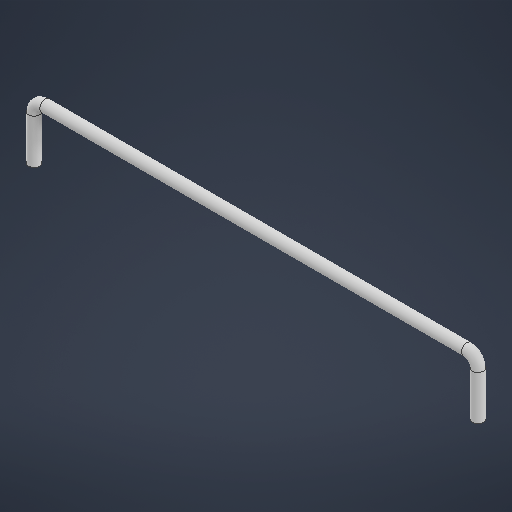
# Autodesk Inventor part: drut
Saved by Autodesk Inventor 2026.2 (Build 302298000, 298)
## iProperties
Created: 2025-12-09
Part Number: drut
Material: Generic
Document SubType Name: Modeling
Designer: janek
Density: 1 g/cm^3
Appearance: Default
Author: janek
Autodesk Inventor part; units mm, degrees
ref_plane "YZ Plane" through (0, 0, 0) normal (1, 0, 0) x (0, 1, 0)
ref_plane "XZ Plane" through (0, 0, 0) normal (0, 1, 0) x (-1, 0, 0)
ref_plane "XY Plane" through (0, 0, 0) normal (0, 0, 1) x (1, 0, 0)
sketch "Sketch1" plane through (0, 0, 0) normal (0, 0, 1) x (1, 0, 0)
  line L0 (0, 0) -> (0, 8)
  line L1 (2, 10) -> (78, 10)
  line L2 (80, 8) -> (80, 0)
  arc A0 (2, 10) -> (0, 8) centre (2, 8) ccw
  arc A1 (80, 8) -> (78, 10) centre (78, 8) ccw
  point P0 (0, 10)
  point P1 (80, 10)
  dimension "d0" = 80
  dimension "d1" = 10
  dimension "d2" = 10
  dimension "d4" = 2
  constraints: 6 end point, 4 point on circle, 4 point on line, 4 tangent, 2 centre point, 2 perpendicular, 1 coincident, 1 equal radius, 1 vertical
  measures "d0" distance of point (0, 10) point (80, 10)
  measures "d1" distance of point (80, 10) L2.end
  measures "d2" distance of L0.start point (0, 10)
  measures "d4" radius of A0
sketch "Sketch2" plane through (0, 0, 0) normal (0, 1, 0) x (-1, 0, 0)
  circle A0 centre (0, 0) radius 1
  dimension "d3" = 2
  constraints: 1 centre point, 1 coincident
  measures "d3" diameter of A0
sweep "Sweep1" add profiles "Sketch2" path "Sketch1"
body "Solid1"
